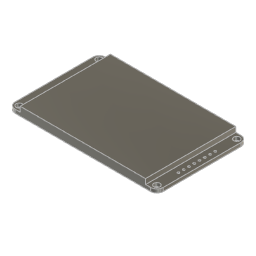
hactar_v9 (Autodesk Fusion 360 archive; units mm, degrees)
design "LCD"
Autodesk Fusion 360 part; units mm, degrees
sketch "Sketch1" plane through (0, 0, 0) normal (0, 0, 1) x (1, 0, 0) in component "2.4\" LCD Module"
  line L0 (0, 0) -> (71, 0)
  line L1 (71, 0) -> (71, 43.3)
  line L2 (71, 43.3) -> (0, 43.3)
  line L3 (0, 43.3) -> (0, 0)
  dimension "d1" = 71
  dimension "d2" = 43.3
  constraint horizontal L0
  constraint vertical L1
  constraint horizontal L2
  constraint vertical L3
  constraint coincident L0.start L3.end
  measures "d1" distance of L0.start L0.end
  measures "d2" distance of L0.start L2.end
extrude "Extrude1" add sketch "Sketch1" along normal blind 1.7 in component "2.4\" LCD Module"
hole "Hole1" at (68.5, 2.5, 1.7) direction (0, 0, -1) diameter 3 depth 5 tip angle 180 in component "2.4\" LCD Module"
hole "Hole2" at (68.5, 40.8, 1.7) direction (0, 0, -1) diameter 3 depth 5 tip angle 180 in component "2.4\" LCD Module"
hole "Hole3" at (2.5, 2.5, 1.7) direction (0, 0, -1) diameter 3 depth 5 tip angle 180 in component "2.4\" LCD Module"
hole "Hole4" at (2.5, 40.8, 1.7) direction (0, 0, -1) diameter 3 depth 5 tip angle 180 in component "2.4\" LCD Module"
fillet "Fillet1" radius 3 4 edges at (71, 0, 0.85) (0, 0, 0.85) (71, 43.3, 0.85) (0, 43.3, 0.85) in component "2.4\" LCD Module"
sketch "Sketch2" plane through (0, 0, 1.7) normal (0, 0, 1) x (-1, 0, 0) in component "2.4\" LCD Module"
  arc A0 (-3, -43.3) -> (0, -40.3) centre (-3, -40.3) ccw
  line L0 (0, -40.3) -> (0, -3)
  arc A1 (0, -3) -> (-3, 0) centre (-3, -3) ccw
  line L1 (-3, 0) -> (-68, 0)
  arc A2 (-68, 0) -> (-71, -3) centre (-68, -3) ccw
  line L2 (-71, -3) -> (-71, -40.3)
  arc A3 (-71, -40.3) -> (-68, -43.3) centre (-68, -40.3) ccw
  line L3 (-68, -43.3) -> (-3, -43.3)
  circle A4 centre (-2.5, -40.8) radius 1.5
  circle A5 centre (-2.5, -2.5) radius 1.5
  circle A6 centre (-68.5, -40.8) radius 1.5
  circle A7 centre (-68.5, -2.5) radius 1.5
  line L4 (-5.4496, 0.0416) -> (-65.5496, 0.0416)
  line L5 (-65.5496, 0.0416) -> (-65.5496, -43.2584)
  line L6 (-65.5496, -43.2584) -> (-5.4496, -43.2584)
  line L7 (-5.4496, -43.2584) -> (-5.4496, 0.0416)
  line L8 (-5.4496, 0.0416) -> (-65.5496, -43.2584) construction
  line L9 (-65.5496, 0.0416) -> (-5.4496, -43.2584) construction
  point P0 (-35.4996, -21.6084)
  dimension "d27" = 60.1
  dimension "d28" = 43.3
  constraint horizontal L4
  constraint perpendicular L4 L5
  constraint parallel L4 L6
  constraint parallel L5 L7
  constraint coincident L8 P0
  constraint coincident L9 P0
  measures "d27" distance of L5.end L6.end
  measures "d28" distance of L4.end L5.end
extrude "Extrude2" add sketch "Sketch2" along normal blind 2.45 contours L1 L5 L6 L7 in component "2.4\" LCD Module"
sketch "Sketch3" plane through (0, 0, 1.7) normal (0, 0, 1) x (-1, 0, 0) in component "2.4\" LCD Module"
  line L0 (-65.5496, -43.2584) -> (-65.5496, 0)
  line L1 (-65.5496, 0) -> (-68, 0)
  arc A0 (-68, 0) -> (-71, -3) centre (-68, -3) ccw
  line L2 (-71, -3) -> (-71, -40.3)
  arc A1 (-71, -40.3) -> (-68, -43.3) centre (-68, -40.3) ccw
  line L3 (-68, -43.3) -> (-3, -43.3)
  arc A2 (-3, -43.3) -> (0, -40.3) centre (-3, -40.3) ccw
  line L4 (0, -40.3) -> (0, -3)
  arc A3 (0, -3) -> (-3, 0) centre (-3, -3) ccw
  line L5 (-3, 0) -> (-5.4496, 0)
  line L6 (-5.4496, 0) -> (-5.4496, -43.2584)
  line L7 (-5.4496, -43.2584) -> (-65.5496, -43.2584)
  circle A4 centre (-2.5, -40.8) radius 1.5
  circle A5 centre (-2.5, -2.5) radius 1.5
  circle A6 centre (-68.5, -40.8) radius 1.5
  circle A7 centre (-68.5, -2.5) radius 1.5
  point P0 (-68.5, -12.7999)
  point P1 (-68.5, -15.3285)
  point P2 (-68.5, -17.857)
  point P3 (-68.5, -20.3856)
  point P4 (-68.5, -22.9142)
  point P5 (-68.5, -25.4427)
  point P6 (-68.5, -27.9713)
  point P7 (-68.5, -30.4999)
  dimension "d33" = 17.7
  dimension "d34" = 0
hole "Hole5" at (68.5, 12.7999, 1.7) at (68.5, 15.3285, 1.7) at (68.5, 17.857, 1.7) at (68.5, 20.3856, 1.7) at (68.5, 22.9142, 1.7) at (68.5, 25.4427, 1.7) at (68.5, 27.9713, 1.7) at (68.5, 30.4999, 1.7) direction (0, 0, -1) diameter 1 depth 5 tip angle 180 in component "2.4\" LCD Module"
sketch "Sketch4" plane through (0, 0, 0) normal (0, 0, -1) x (1, 0, 0) in component "2.4\" LCD Module"
  circle A0 centre (68.5, -27.9713) radius 0.5
  circle A1 centre (68.5, -22.9142) radius 0.5
  circle A2 centre (68.5, -17.857) radius 0.5
  circle A3 centre (68.5, -12.7999) radius 0.5
  circle A4 centre (68.5, -15.3285) radius 0.5
  circle A5 centre (68.5, -20.3856) radius 0.5
  circle A6 centre (68.5, -25.4427) radius 0.5
  circle A7 centre (68.5, -30.4999) radius 0.5
  circle A8 centre (2.5, -40.8) radius 1.5
  circle A9 centre (2.5, -2.5) radius 1.5
  circle A10 centre (68.5, -40.8) radius 1.5
  circle A11 centre (68.5, -2.5) radius 1.5
  arc A12 (0, -40.3) -> (3, -43.3) centre (3, -40.3) ccw
  line L0 (3, -43.3) -> (68, -43.3)
  arc A13 (68, -43.3) -> (71, -40.3) centre (68, -40.3) ccw
  line L1 (71, -40.3) -> (71, -3)
  arc A14 (71, -3) -> (68, 0) centre (68, -3) ccw
  line L2 (68, 0) -> (3, 0)
  arc A15 (3, 0) -> (0, -3) centre (3, -3) ccw
  line L3 (0, -3) -> (0, -40.3)
  line L4 (12.6, -31.65) -> (5, -31.65)
  line L5 (5, -31.65) -> (5, -11.65)
  line L6 (5, -11.65) -> (12.6, -11.65)
  line L7 (12.6, -11.65) -> (12.6, -31.65)
  dimension "d38" = 7.6
  dimension "d39" = 20
  constraint horizontal L4
  constraint vertical L5
  constraint horizontal L6
  constraint vertical L7
  measures "d38" distance of L4.start L4.end
  measures "d39" distance of L4.start L6.end
extrude "Extrude3" add sketch "Sketch4" along normal blind 5.52 contours L4 L5 L6 L7 in component "2.4\" LCD Module"
component "2.4\" LCD Module" placed x (1, 0, 0) y (0, 1, 0) z (0, 0, 1) at (0, 0, 0)

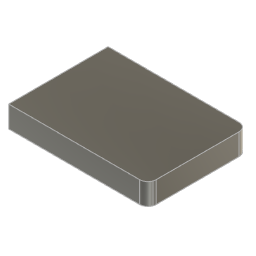
design "LP653042"
Autodesk Fusion 360 part; units mm, degrees
sketch "Sketch1" plane through (0, 0, 0) normal (0, 0, 1) x (1, 0, 0) in component "LP653042"
  line L0 (0, 0) -> (42, 0)
  line L1 (42, 0) -> (42, 30)
  line L2 (42, 30) -> (0, 30)
  line L3 (0, 30) -> (0, 0)
  dimension "d1" = 42
  dimension "d2" = 30
  constraint horizontal L0
  constraint vertical L1
  constraint horizontal L2
  constraint vertical L3
  constraint coincident L0.start L3.end
  measures "d1" distance of L0.start L0.end
  measures "d2" distance of L0.start L2.end
extrude "Extrude1" add sketch "Sketch1" along normal blind 6.5 in component "LP653042"
fillet "Fillet1" radius 2.5 2 edges at (42, 0, 3.25) (42, 30, 3.25) in component "LP653042"
component "LP653042" placed x (1, 0, 0) y (0, 1, 0) z (0, 0, 1) at (0, 0, 0)

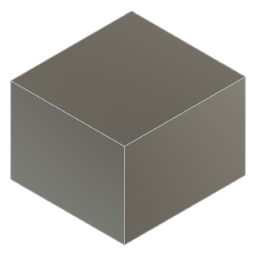
design "BatteryConnector"
Autodesk Fusion 360 part; units mm, degrees
sketch "Sketch1" plane through (0, 0, 0) normal (0, 0, 1) x (1, 0, 0) in component "Connector"
  line L0 (4, 4.25) -> (-4, 4.25)
  line L1 (-4, 4.25) -> (-4, -4.25)
  line L2 (-4, -4.25) -> (4, -4.25)
  line L3 (4, -4.25) -> (4, 4.25)
  line L4 (4, 4.25) -> (-4, -4.25) construction
  line L5 (-4, 4.25) -> (4, -4.25) construction
  dimension "d1" = 8
  dimension "d2" = 8.5
  constraint horizontal L0
  constraint perpendicular L0 L1
  constraint parallel L0 L2
  constraint parallel L1 L3
  constraint coincident L4 origin
  constraint coincident L5 origin
  measures "d1" distance of L1.end L2.end
  measures "d2" distance of L0.end L1.end
extrude "Extrude1" add sketch "Sketch1" along normal blind 6 in component "Connector"
component "Connector" placed x (1, 0, 0) y (0, 1, 0) z (0, 0, 1) at (0, 0, 0)

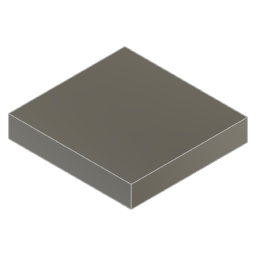
design "WifiChip"
Autodesk Fusion 360 part; units mm, degrees
sketch "Sketch1" plane through (0, 0, 0) normal (0, 0, 1) x (1, 0, 0) in component "Chip"
  line L0 (9.6, 9.1) -> (-9.6, 9.1)
  line L1 (-9.6, 9.1) -> (-9.6, -9.1)
  line L2 (-9.6, -9.1) -> (9.6, -9.1)
  line L3 (9.6, -9.1) -> (9.6, 9.1)
  line L4 (9.6, 9.1) -> (-9.6, -9.1) construction
  line L5 (-9.6, 9.1) -> (9.6, -9.1) construction
  dimension "d1" = 19.2
  dimension "d2" = 18.2
  constraint horizontal L0
  constraint perpendicular L0 L1
  constraint parallel L0 L2
  constraint parallel L1 L3
  constraint coincident L4 origin
  constraint coincident L5 origin
  measures "d1" distance of L1.end L2.end
  measures "d2" distance of L0.end L1.end
extrude "Extrude1" add sketch "Sketch1" along normal blind 3.4 in component "Chip"
component "Chip" placed x (1, 0, 0) y (0, 1, 0) z (0, 0, 1) at (0, 0, 0)
